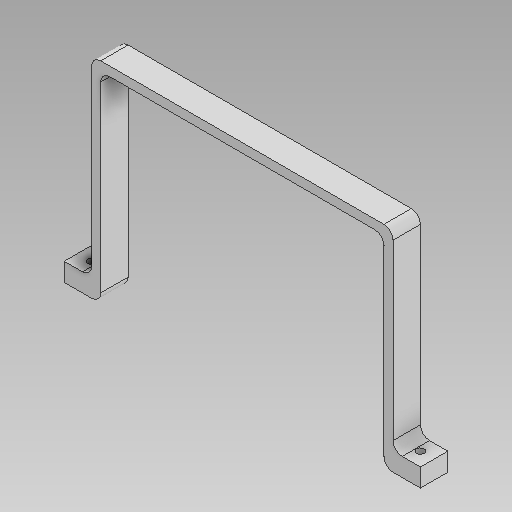
# Autodesk Inventor part: Box_clamp
Saved by Autodesk Inventor 2026.1 (Build 301233000, 233)
## iProperties
Created: 2026-02-06
Part Number: Box_clamp
Material: Generic
Document SubType Name: Modeling
Designer: aleja
Density: 1 g/cm^3
Appearance: Default
Author: aleja
Autodesk Inventor part; units mm, degrees
ref_plane "YZ Plane" through (0, 0, 0) normal (1, 0, 0) x (0, 1, 0)
ref_plane "XZ Plane" through (0, 0, 0) normal (0, 1, 0) x (-1, 0, 0)
ref_plane "XY Plane" through (0, 0, 0) normal (0, 0, 1) x (1, 0, 0)
sketch "Sketch1" plane through (0, 0, 0) normal (0, 1, 0) x (-1, 0, 0)
  line L0 (0, 0) -> (5, 0)
  line L1 (5, 0) -> (5, -115)
  line L2 (5, -115) -> (0, -115)
  line L3 (0, -115) -> (0, 0)
  line L4 (5, -115) -> (20, -115)
  line L5 (20, -115) -> (20, -105)
  line L6 (20, -105) -> (5, -105)
  line L7 (5, -105) -> (5, -115)
  line L8 (0, -10) -> (0, 0)
  point P0 (5, -105)
  dimension "d0" = 5
  dimension "d1" = 115
  dimension "d2" = 15
  dimension "d3" = 10
  constraints: 18 end point, 4 parallel, 2 horizontal, 2 perpendicular
  measures "d0" distance of L1.end L2.end
  measures "d1" distance of L0.end L1.end
  measures "d2" distance of L6.end L5.end
  measures "d3" distance of L5.end L4.end
extrude "Extrusion1" add sketch "Sketch1" along normal blind 15
sketch "Sketch6" plane through (0, 0, 0) normal (1, 0, 0) x (0, 0, -1)
  line L0 (105, 0) -> (0, 0) projected
  line L1 (0, 0) -> (5, 0)
  line L2 (5, 0) -> (5, 15)
  line L3 (5, 15) -> (0, 15)
  line L4 (0, 15) -> (0, 0)
  dimension "d24" = 5
  dimension "d25" = 15
  constraints: 8 end point, 2 parallel, 1 horizontal, 1 perpendicular
  measures "d24" distance of L3.end L2.end
  measures "d25" distance of L2.end L1.end
extrude "Extrusion4" add sketch "Sketch6" along normal blind 77.5
sketch "Sketch7" plane through (0, 0, 0) normal (0, -1, 0) x (1, 0, 0)
  line L0 (-20, -105) -> (-5, -105) projected
  line L1 (-20, -115) -> (-20, -105) projected
  line L2 (0, -115) -> (-20, -115) projected
  line L3 (0, -5) -> (0, -115) projected
  line L4 (0, -5) -> (77.5, -5) projected
  line L5 (77.5, 0) -> (77.5, -5) projected
  line L6 (-5, 0) -> (77.5, 0) projected
  line L7 (-5, -105) -> (-5, 0) projected
  line L8 (175, -105) -> (160, -105)
  line L9 (175, -115) -> (175, -105)
  line L10 (155, -115) -> (175, -115)
  line L11 (155, -5) -> (155, -115)
  line L12 (155, -5) -> (77.5, -5)
  line L13 (160, 0) -> (77.5, 0)
  line L14 (160, -105) -> (160, 0)
  point P0 (0, 0)
  constraints: 14 end point, 6 symmetric about line
extrude "Extrusion5" add sketch "Sketch7" against normal up to surface (15 mm away) contours L13 L14 L8 L9 L10 L11 L12 L5
sketch "Sketch2" plane through (-20, 0, -105) normal (0, 0, 1) x (1, 0, 0)
  line L0 (0, 0) -> (0, 15) projected
  circle A0 centre (7.5, 7.5) radius 2.15
  line L1 (7.5, 7.5) -> (0, 7.5) construction
  line L2 (15, 15) -> (180, 15) projected
  line L3 (97.5, 15) -> (97.5, 37.3705) construction
  circle A1 centre (187.5, 7.5) radius 2.15
  point P0 (20, 0)
  dimension "d8" = 4.3
  dimension "d20" = 7.5
  constraints: 4 end point, 2 centre point, 2 midpoint, 1 symmetric about line, 1 vertical, 1 other
  measures "d8" diameter of A0
  measures "d20" distance of L1.start L1.end
extrude "Extrusion2" cut sketch "Sketch2" against normal blind 15
fillet "Fillet2" radius 5 8 edges at (0, 7.5, -5) (0, 7.5, -115) (155, 7.5, -115) (160, 7.5, 0) (155, 7.5, -5) (-5, 7.5, 0) (-5, 7.5, -105) (160, 7.5, -105)
body "Solid1"
